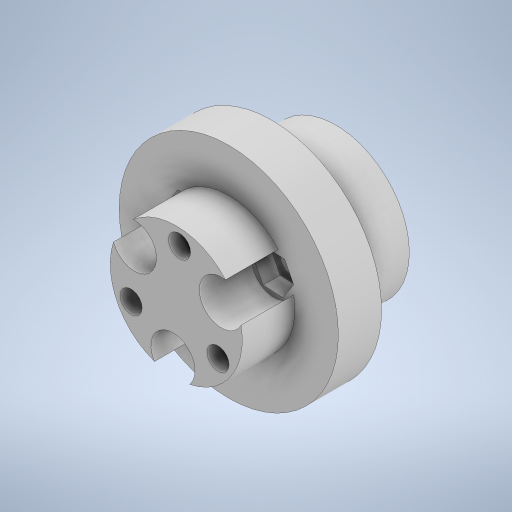
# Autodesk Inventor part: Os
Saved by Autodesk Inventor 2023 (Build 270158000, 158)
## iProperties
Created: 2023-01-20
Part Number: Os
Material: Generic
Document SubType Name: Modeling
Designer: Kamil
Density: 1 g/cm^3
Appearance: Default
Mass: 24.6668 g
Surface Area: 88.8395 cm^2
Volume: 24.6668 cm^3
Author: Kamil
Autodesk Inventor part; units mm, degrees
ref_plane "YZ Plane" through (0, 0, 0) normal (1, 0, 0) x (0, 1, 0)
ref_plane "XZ Plane" through (0, 0, 0) normal (0, 1, 0) x (-1, 0, 0)
ref_plane "XY Plane" through (0, 0, 0) normal (0, 0, 1) x (1, 0, 0)
sketch "Sketch1" plane through (0, 0, 0) normal (0, 0, 1) x (1, 0, 0)
  circle A0 centre (0, 0) radius 23.3333 projected
  arc A1 (-39.2843, 4.1223) -> (-36.4252, -2.8784) centre (-31.328, 3.2874) ccw projected
  arc A2 (-35.6202, -8.1415) -> (-36.4252, -2.8784) centre (-38.9739, -5.9614) ccw projected
  arc A3 (-35.6202, -8.1415) -> (-36.2558, -15.6768) centre (-28.9129, -12.5018) ccw projected
  arc A4 (-36.2558, -15.6768) -> (33.8969, -20.2792) centre (0, 0) ccw projected
  arc A5 (33.8969, -20.2792) -> (34.2512, -12.7254) centre (27.0317, -16.172) ccw projected
  arc A6 (35.737, -7.6127) -> (34.2512, -12.7254) centre (37.861, -11.0021) ccw projected
  arc A7 (35.737, -7.6127) -> (39.4862, -1.0454) centre (31.489, -0.8337) ccw projected
  arc A8 (39.4862, -1.0454) -> (-39.2843, 4.1223) centre (0, 0) ccw projected
  circle A9 centre (-9.1932, -4.5329) radius 2 projected
  circle A10 centre (9.1932, 4.5329) radius 2 projected
  circle A11 centre (-0.671, -10.228) radius 2 projected
  circle A12 centre (-8.5222, 5.6951) radius 2 projected
  circle A13 centre (0.671, 10.228) radius 2 projected
  circle A14 centre (8.5222, -5.6951) radius 2 projected
  circle A15 centre (0, 0) radius 13.4591 projected
  line L0 (-5.9382, 0.859) -> (-7.1311, 0.7284) projected
  arc A16 (-5.6118, -2.1232) -> (-5.9382, 0.859) centre (0, 0) ccw projected
  line L1 (-6.8047, -2.2538) -> (-5.6118, -2.1232) projected
  line L2 (-7.1311, 0.7284) -> (-6.8047, -2.2538) projected
  line L3 (23.3333, 0) -> (22.3333, 0)
  circle A17 centre (0, 0) radius 22.3333
  circle A18 centre (0, 0) radius 6
  circle A19 centre (16.7628, -26.571) radius 3.75 projected
  circle A20 centre (-29.1794, 11.6435) radius 3.75 projected
  circle A21 centre (2.0567, 31.3493) radius 3.75 projected
  circle A22 centre (-20.0905, -24.1532) radius 3.75 projected
  circle A23 centre (30.4505, 7.7314) radius 3.75 projected
  point P0 (0, 0)
  dimension "d0" = 1
  constraints: 2 coincident, 2 end point, 2 horizontal alignment, 1 horizontal, 6 other
  measures "d0" distance of L3.start L3.end
extrude "Extrusion1" add sketch "Sketch1" along normal blind 3.8 contours A15 | A18 L1 L2 L0 | A16 A18 | A17
sketch "Sketch2" plane through (0, 0, 0) normal (0, 0, -1) x (-1, 0, 0)
  circle A0 centre (0, 0) radius 15 projected
  circle A1 centre (0, 0) radius 22.3333 projected
  circle A2 centre (9.1932, -4.5329) radius 2 projected
  circle A3 centre (-9.1932, 4.5329) radius 2 projected
  circle A4 centre (0.671, -10.228) radius 2 projected
  circle A5 centre (8.5222, 5.6951) radius 2 projected
  circle A6 centre (-0.671, 10.228) radius 2 projected
  circle A7 centre (-8.5222, -5.6951) radius 2 projected
  point P0 (0, 0)
ref_plane "Work Plane1" through (-21.6708, -21.6708, -13) normal (0, 0, -1) x (0, 1, 0)
extrude "Extrusion2" add sketch "Sketch2" along normal up to surface (13 mm away) contours A0
sketch "Sketch3" plane through (0, 0, 3.8) normal (0, 0, 1) x (1, 0, 0)
  point P0 (0, 0)
sketch "Sketch4" plane through (0, 0, -13) normal (0, 0, -1) x (-1, 0, 0)
  circle A0 centre (0, 0) radius 15 projected
  circle A1 centre (-8.5222, -5.6951) radius 2 projected
  circle A2 centre (-0.671, 10.228) radius 2 projected
  circle A3 centre (8.5222, 5.6951) radius 2 projected
  circle A4 centre (0.671, -10.228) radius 2 projected
  circle A5 centre (-9.1932, 4.5329) radius 2 projected
  circle A6 centre (9.1932, -4.5329) radius 2 projected
  line L0 (0, 0) -> (9.1932, -4.5329)
  line L1 (9.1932, -4.5329) -> (12.3324, -6.0807)
  circle A7 centre (9.1932, -4.5329) radius 2 projected
  circle A8 centre (9.1932, -4.5329) radius 3.5
  circle A9 centre (8.5222, 5.6951) radius 3.5
  circle A10 centre (-0.671, 10.228) radius 3.5
  circle A11 centre (-9.1932, 4.5329) radius 3.5
  circle A12 centre (-8.5222, -5.6951) radius 3.5
  circle A13 centre (0.671, -10.228) radius 3.5
  point P0 (0, 0)
  point P1 (11.4322, 7.6398)
  point P2 (-0.9001, 13.7205)
  point P3 (-12.3324, 6.0807)
  point P4 (-11.4322, -7.6398)
  point P5 (0.9001, -13.7205)
  dimension "d5" = 3.5
  dimension "d8" = 360
  constraints: 4 end point, 1 coincident, 1 collinear, 37 other
  measures "d5" distance of L0.end L1.end
extrude "Extrusion3" cut sketch "Sketch4" against normal blind 5 contours A1 | A6 L1 L0 | A6 L0 A8 L1 | L0 L1 A6 | A6 L1 A8 L0 | A10 | A12
sketch "Sketch5" plane through (0, 0, 3.8) normal (0, 0, 1) x (1, 0, 0)
  circle A0 centre (0, 0) radius 22.3333 projected
  circle A1 centre (-9.1932, -4.5329) radius 2 projected
  circle A2 centre (9.1932, 4.5329) radius 2 projected
  circle A3 centre (-0.671, -10.228) radius 2 projected
  circle A4 centre (-8.5222, 5.6951) radius 2 projected
  circle A5 centre (0.671, 10.228) radius 2 projected
  circle A6 centre (8.5222, -5.6951) radius 2 projected
  line L0 (0, 0) -> (-0.671, -10.228)
  circle A7 centre (-0.671, -10.228) radius 2 projected
  line L1 (-0.671, -10.228) -> (-1.462, -22.2854)
  circle A8 centre (0, 0) radius 22.3333 projected
  line L2 (-0.671, -10.228) -> (-0.9001, -13.7205)
  line L3 (-3.0871, -13.8731) -> (-5.0083, -9.9765)
  line L4 (-5.0083, -9.9765) -> (-2.5944, -6.3644)
  line L5 (-2.5944, -6.3644) -> (1.7407, -6.6488)
  line L6 (1.7407, -6.6488) -> (3.662, -10.5454)
  line L7 (3.662, -10.5454) -> (1.2481, -14.1575)
  line L8 (1.2481, -14.1575) -> (-3.0871, -13.8731)
  line L9 (4.2145, -5.429) -> (6.6284, -1.8169)
  line L10 (6.1358, -9.3256) -> (4.2145, -5.429)
  line L11 (10.4709, -9.61) -> (6.1358, -9.3256)
  line L12 (12.8848, -5.9979) -> (10.4709, -9.61)
  line L13 (10.9635, -2.1013) -> (12.8848, -5.9979)
  line L14 (6.6284, -1.8169) -> (10.9635, -2.1013)
  line L15 (6.8089, 0.9353) -> (4.8877, 4.8319)
  line L16 (11.1441, 0.6509) -> (6.8089, 0.9353)
  line L17 (13.558, 4.2631) -> (11.1441, 0.6509)
  line L18 (11.6367, 8.1596) -> (13.558, 4.2631)
  line L19 (7.3016, 8.4441) -> (11.6367, 8.1596)
  line L20 (4.8877, 4.8319) -> (7.3016, 8.4441)
  line L21 (2.5944, 6.3644) -> (-1.7407, 6.6488)
  line L22 (5.0083, 9.9765) -> (2.5944, 6.3644)
  line L23 (3.0871, 13.8731) -> (5.0083, 9.9765)
  line L24 (-1.2481, 14.1575) -> (3.0871, 13.8731)
  line L25 (-3.662, 10.5454) -> (-1.2481, 14.1575)
  line L26 (-1.7407, 6.6488) -> (-3.662, 10.5454)
  line L27 (-4.2145, 5.429) -> (-6.6284, 1.8169)
  line L28 (-6.1358, 9.3256) -> (-4.2145, 5.429)
  line L29 (-10.4709, 9.61) -> (-6.1358, 9.3256)
  line L30 (-12.8848, 5.9979) -> (-10.4709, 9.61)
  line L31 (-10.9635, 2.1013) -> (-12.8848, 5.9979)
  line L32 (-6.6284, 1.8169) -> (-10.9635, 2.1013)
  line L33 (-6.8089, -0.9353) -> (-4.8877, -4.8319)
  line L34 (-11.1441, -0.6509) -> (-6.8089, -0.9353)
  line L35 (-13.558, -4.2631) -> (-11.1441, -0.6509)
  line L36 (-11.6367, -8.1596) -> (-13.558, -4.2631)
  line L37 (-7.3016, -8.4441) -> (-11.6367, -8.1596)
  line L38 (-4.8877, -4.8319) -> (-7.3016, -8.4441)
  point P0 (0, 0)
  point P1 (-0.6732, -10.261)
  point P2 (-0.9195, -14.0153)
  point P3 (11.6779, -7.8039)
  point P4 (12.5974, 6.2114)
  point P5 (0.9195, 14.0153)
  point P6 (-11.6779, 7.8039)
  point P7 (-12.5974, -6.2114)
  dimension "d13" = 3.5
  dimension "d16" = 360
  constraints: 78 end point, 2 point on line, 1 collinear, 1 midpoint, 94 other
  measures "d13" distance of L1.start L2.end
extrude "Extrusion4" add sketch "Sketch5" along normal blind 5 contours A0 | L9 L14 L13 L12 L11 L10 | L21 L26 L25 L24 L23 L22 | L33 L38 L37 L36 L35 L34
sketch "Sketch6" plane through (0, 0, 3.8) normal (0, 0, 1) x (1, 0, 0)
  line L0 (6.8089, 0.9353) -> (11.1441, 0.6509) projected
  line L1 (11.1441, 0.6509) -> (13.558, 4.2631) projected
  line L2 (13.558, 4.2631) -> (11.6367, 8.1596) projected
  line L3 (11.6367, 8.1596) -> (7.3016, 8.4441) projected
  line L4 (7.3016, 8.4441) -> (4.8877, 4.8319) projected
  line L5 (4.8877, 4.8319) -> (6.8089, 0.9353) projected
  circle A0 centre (9.1932, 4.5329) radius 2 projected
  circle A1 centre (0, 0) radius 22.3333 projected
  circle A2 centre (8.5222, -5.6951) radius 2 projected
  circle A3 centre (0.671, 10.228) radius 2 projected
  circle A4 centre (-9.1932, -4.5329) radius 2 projected
  line L6 (1.2481, -14.1575) -> (-3.0871, -13.8731) projected
  line L7 (-3.0871, -13.8731) -> (-5.0083, -9.9765) projected
  line L8 (-5.0083, -9.9765) -> (-2.5944, -6.3644) projected
  line L9 (-2.5944, -6.3644) -> (1.7407, -6.6488) projected
  line L10 (1.7407, -6.6488) -> (3.662, -10.5454) projected
  line L11 (3.662, -10.5454) -> (1.2481, -14.1575) projected
  line L12 (-4.2145, 5.429) -> (-6.6284, 1.8169) projected
  line L13 (-6.6284, 1.8169) -> (-10.9635, 2.1013) projected
  line L14 (-10.9635, 2.1013) -> (-12.8848, 5.9979) projected
  line L15 (-12.8848, 5.9979) -> (-10.4709, 9.61) projected
  line L16 (-10.4709, 9.61) -> (-6.1358, 9.3256) projected
  line L17 (-6.1358, 9.3256) -> (-4.2145, 5.429) projected
  line L18 (6.8089, 0.9353) -> (4.8877, 4.8319) projected
  line L19 (4.8877, 4.8319) -> (7.3016, 8.4441) projected
  line L20 (7.3016, 8.4441) -> (11.6367, 8.1596) projected
  line L21 (11.6367, 8.1596) -> (13.558, 4.2631) projected
  line L22 (13.558, 4.2631) -> (11.1441, 0.6509) projected
  line L23 (11.1441, 0.6509) -> (6.8089, 0.9353) projected
  circle A5 centre (-0.671, -10.228) radius 2 projected
  circle A6 centre (-8.5222, 5.6951) radius 2 projected
  point P0 (0, 0)
extrude "Extrusion5" add sketch "Sketch6" along normal blind 1.5 contours L5 L4 L3 L2 L1 L0 | L6 L7 L8 L9 L10 L11 | L12 L13 L14 L15 L16 L17
sketch "Sketch7" plane through (0, 0, 8.8) normal (0, 0, 1) x (1, 0, 0)
  circle A0 centre (8.5222, -5.6951) radius 2 projected
  circle A1 centre (9.1932, 4.5329) radius 2 projected
  circle A2 centre (-0.671, -10.228) radius 2 projected
  circle A3 centre (0.671, 10.228) radius 2 projected
  circle A4 centre (-9.1932, -4.5329) radius 2 projected
  arc A5 (5.9995, 0.0758) -> (5.2863, -2.8382) centre (0, 0) ccw projected
  line L0 (7.1651, -0.2095) -> (5.9995, 0.0758) projected
  line L1 (6.4519, -3.1235) -> (7.1651, -0.2095) projected
  line L2 (5.2863, -2.8382) -> (6.4519, -3.1235) projected
  circle A6 centre (-8.5222, 5.6951) radius 2 projected
  circle A7 centre (0, 0) radius 13.4542 projected
  circle A8 centre (0, 0) radius 6
  circle A9 centre (0, 0) radius 22.3333 projected
  circle A10 centre (8.5222, -5.6951) radius 2 projected
  circle A11 centre (0.671, 10.228) radius 2 projected
  circle A12 centre (-9.1932, -4.5329) radius 2 projected
  line L3 (1.2481, -14.1575) -> (-3.0871, -13.8731) projected
  line L4 (-3.0871, -13.8731) -> (-5.0083, -9.9765) projected
  line L5 (-5.0083, -9.9765) -> (-2.5944, -6.3644) projected
  line L6 (-2.5944, -6.3644) -> (1.7407, -6.6488) projected
  line L7 (1.7407, -6.6488) -> (3.662, -10.5454) projected
  line L8 (3.662, -10.5454) -> (1.2481, -14.1575) projected
  line L9 (-4.2145, 5.429) -> (-6.6284, 1.8169) projected
  line L10 (-6.6284, 1.8169) -> (-10.9635, 2.1013) projected
  line L11 (-10.9635, 2.1013) -> (-12.8848, 5.9979) projected
  line L12 (-12.8848, 5.9979) -> (-10.4709, 9.61) projected
  line L13 (-10.4709, 9.61) -> (-6.1358, 9.3256) projected
  line L14 (-6.1358, 9.3256) -> (-4.2145, 5.429) projected
  line L15 (6.8089, 0.9353) -> (4.8877, 4.8319) projected
  line L16 (4.8877, 4.8319) -> (7.3016, 8.4441) projected
  line L17 (7.3016, 8.4441) -> (11.6367, 8.1596) projected
  line L18 (11.6367, 8.1596) -> (13.558, 4.2631) projected
  line L19 (13.558, 4.2631) -> (11.1441, 0.6509) projected
  line L20 (11.1441, 0.6509) -> (6.8089, 0.9353) projected
  point P0 (0, 0)
  point P1 (1.7989, -13.3334)
  point P2 (13.0072, 3.4389)
  point P3 (10.6476, 8.2245)
  point P4 (-9.4818, 9.5451)
  point P5 (-12.4465, 5.1088)
  point P6 (-3.5254, -12.9841)
  point P7 (5.9995, 0.0758)
  constraints: 1 coincident, 3 other
extrude "Extrusion6" add sketch "Sketch7" along normal blind 5.2 contours L0 L1 L2 A8 | A7 L8 L7 L6 L5 L4 L11 L10 L9 L14 L13 L17 L16 L15 L20 L19
sketch "Sketch8" plane through (0, 0, 8.8) normal (0, 0, 1) x (1, 0, 0)
  circle A0 centre (0, 0) radius 6 projected
  point P0 (0, 0)
extrude "Extrusion7" add sketch "Sketch8" along normal up to surface (5.2 mm away)
sketch "Sketch9" plane through (0, 0, 14) normal (0, 0, 1) x (1, 0, 0)
  line L0 (3.662, -10.5454) -> (1.7989, -13.3334) projected
  arc A0 (1.7989, -13.3334) -> (13.0072, 3.4389) centre (0, 0) ccw projected
  line L1 (13.0072, 3.4389) -> (11.1441, 0.6509) projected
  line L2 (11.1441, 0.6509) -> (6.8089, 0.9353) projected
  line L3 (6.8089, 0.9353) -> (4.8877, 4.8319) projected
  line L4 (4.8877, 4.8319) -> (7.3016, 8.4441) projected
  line L5 (7.3016, 8.4441) -> (10.6476, 8.2245) projected
  arc A1 (10.6476, 8.2245) -> (-9.4818, 9.5451) centre (0, 0) ccw projected
  line L6 (-9.4818, 9.5451) -> (-6.1358, 9.3256) projected
  line L7 (-6.1358, 9.3256) -> (-4.2145, 5.429) projected
  line L8 (-4.2145, 5.429) -> (-6.6284, 1.8169) projected
  line L9 (-6.6284, 1.8169) -> (-10.9635, 2.1013) projected
  line L10 (-10.9635, 2.1013) -> (-12.4465, 5.1088) projected
  arc A2 (-12.4465, 5.1088) -> (-3.5254, -12.9841) centre (0, 0) ccw projected
  line L11 (-3.5254, -12.9841) -> (-5.0083, -9.9765) projected
  line L12 (-5.0083, -9.9765) -> (-2.5944, -6.3644) projected
  line L13 (-2.5944, -6.3644) -> (1.7407, -6.6488) projected
  line L14 (1.7407, -6.6488) -> (3.662, -10.5454) projected
  circle A3 centre (8.5222, -5.6951) radius 2 projected
  circle A4 centre (0.671, 10.228) radius 2 projected
  circle A5 centre (-9.1932, -4.5329) radius 2 projected
  point P0 (0, 0)
extrude "Extrusion8" add sketch "Sketch9" along normal blind 5.5
fillet "Fillet2" radius 0.4 12 edges at (-4.2669, -11.4803, 19.5) (-3.5254, -12.9841, 14.15) (2.7304, -11.9394, 19.5) (1.7989, -13.3334, 14.15) (12.0757, 2.0449, 19.5) (13.0072, 3.4389, 14.15) (8.9746, 8.3343, 19.5) (10.6476, 8.2245, 14.15) (-7.8088, 9.4354, 19.5) (-9.4818, 9.5451, 14.15) (-11.705, 3.6051, 19.5) (-12.4465, 5.1088, 14.15)
sketch "Sketch10" plane through (0, 0, 19.5) normal (0, 0, 1) x (1, 0, 0)
  line L0 (-12.5711, 4.457) -> (-11.4244, 2.1315) projected
  line L1 (-5.265, -10.3606) -> (-4.1183, -12.686) projected
  line L2 (-5.265, -10.3606) -> (-2.5944, -6.3644) projected
  line L3 (-2.5944, -6.3644) -> (1.7407, -6.6488) projected
  line L4 (1.7407, -6.6488) -> (3.8663, -10.9596) projected
  line L5 (2.4256, -13.1154) -> (3.8663, -10.9596) projected
  line L6 (11.605, 0.6207) -> (13.0456, 2.7764) projected
  line L7 (11.605, 0.6207) -> (6.8089, 0.9353) projected
  line L8 (6.8089, 0.9353) -> (4.8877, 4.8319) projected
  line L9 (4.8877, 4.8319) -> (7.5582, 8.8281) projected
  line L10 (10.1454, 8.6583) -> (7.5582, 8.8281) projected
  line L11 (-6.34, 9.7399) -> (-8.9273, 9.9096) projected
  line L12 (-6.34, 9.7399) -> (-4.2145, 5.429) projected
  line L13 (-4.2145, 5.429) -> (-6.6284, 1.8169) projected
  line L14 (-6.6284, 1.8169) -> (-11.4244, 2.1315) projected
  circle A0 centre (-9.1932, -4.5329) radius 2 projected
  circle A1 centre (0.671, 10.228) radius 2 projected
  circle A2 centre (8.5222, -5.6951) radius 2 projected
  circle A3 centre (-8.5222, 5.6951) radius 2 projected
  circle A4 centre (-0.671, -10.228) radius 2 projected
  circle A5 centre (9.1932, 4.5329) radius 2 projected
  circle A6 centre (-8.5222, 5.6951) radius 2.25
  circle A7 centre (0.671, 10.228) radius 2 projected
  circle A8 centre (0.671, 10.228) radius 2.25
  circle A9 centre (9.1932, 4.5329) radius 2.25
  circle A10 centre (-0.671, -10.228) radius 2.25
  circle A11 centre (8.5222, -5.6951) radius 2 projected
  circle A12 centre (8.5222, -5.6951) radius 2.25
  circle A13 centre (-9.1932, -4.5329) radius 2 projected
  circle A14 centre (-9.1932, -4.5329) radius 2.25
  arc A15 (-12.5711, 4.457) -> (-12.7739, 4.2238) centre (-12.3942, 4.0983) ccw projected
  arc A16 (-12.7739, 4.2238) -> (-4.4268, -12.705) centre (0, 0) ccw projected
  arc A17 (-4.4268, -12.705) -> (-4.1183, -12.686) centre (-4.2952, -12.3273) ccw projected
  arc A18 (2.4256, -13.1154) -> (2.729, -13.1745) centre (2.6479, -12.7828) ccw projected
  arc A19 (2.729, -13.1745) -> (13.2163, 2.5187) centre (0, 0) ccw projected
  arc A20 (13.2163, 2.5187) -> (13.0456, 2.7764) centre (12.8234, 2.4439) ccw projected
  arc A21 (10.1454, 8.6583) -> (10.0449, 8.9506) centre (9.7463, 8.6845) ccw projected
  arc A22 (10.0449, 8.9506) -> (-8.7894, 10.1863) centre (0, 0) ccw projected
  arc A23 (-8.7894, 10.1863) -> (-8.9273, 9.9096) centre (-8.5281, 9.8834) ccw projected
  point P0 (0, 0)
  dimension "d30" = 4.5
  dimension "d31" = 4.5
  dimension "d32" = 4.5
  dimension "d33" = 4.5
  dimension "d34" = 4.5
  dimension "d35" = 4.5
  constraints: 6 centre point, 5 coincident
  measures "d30" diameter of A6
  measures "d31" diameter of A8
  measures "d32" diameter of A9
  measures "d33" diameter of A10
  measures "d34" diameter of A12
  measures "d35" diameter of A14
extrude "Extrusion9" cut sketch "Sketch10" against normal through all contours A0 | A1 | A2 | A3 | A4 | A5 | A6 | A8 | A9 | A10 | A12 | A14
sketch "Sketch12" plane through (-9.1932, -4.5329, -8) normal (0, 0, -1) x (-1, 0, 0)
  circle A0 centre (-8.5222, -5.6951) radius 2.25 projected
  circle A1 centre (-0.671, 10.228) radius 2.25 projected
  circle A2 centre (-18.3864, 9.0658) radius 2.25 projected
  circle A3 centre (-9.8642, 14.7609) radius 3.5 projected
  circle A4 centre (-17.7154, -1.1622) radius 3.5 projected
  circle A5 centre (0, 0) radius 3.5 projected
  circle A6 centre (-9.1932, 4.5329) radius 15 projected
  point P0 (-9.1932, 4.5329)
extrude "Extrusion11" cut sketch "Sketch12" against normal blind 3 contours A3 | A4 | A5
sketch "Szkic15" plane through (0, 0, 5.3) normal (0, 0, 1) x (1, 0, 0)
  circle A0 centre (-8.5222, 5.6951) radius 2.25 projected
  line L0 (-10.4709, 9.61) -> (-6.1358, 9.3256) projected
  line L1 (-12.8848, 5.9979) -> (-10.4709, 9.61) projected
  line L2 (-10.9635, 2.1013) -> (-12.8848, 5.9979) projected
  line L3 (-6.6284, 1.8169) -> (-10.9635, 2.1013) projected
  line L4 (-4.2145, 5.429) -> (-6.6284, 1.8169) projected
  line L5 (-6.1358, 9.3256) -> (-4.2145, 5.429) projected
  circle A1 centre (-0.671, -10.228) radius 2.25 projected
  line L6 (1.7407, -6.6488) -> (3.662, -10.5454) projected
  line L7 (-2.5944, -6.3644) -> (1.7407, -6.6488) projected
  line L8 (-5.0083, -9.9765) -> (-2.5944, -6.3644) projected
  line L9 (-3.0871, -13.8731) -> (-5.0083, -9.9765) projected
  line L10 (1.2481, -14.1575) -> (-3.0871, -13.8731) projected
  line L11 (3.662, -10.5454) -> (1.2481, -14.1575) projected
  circle A2 centre (9.1932, 4.5329) radius 2.25 projected
  line L12 (11.1441, 0.6509) -> (6.8089, 0.9353) projected
  line L13 (13.558, 4.2631) -> (11.1441, 0.6509) projected
  line L14 (11.6367, 8.1596) -> (13.558, 4.2631) projected
  line L15 (7.3016, 8.4441) -> (11.6367, 8.1596) projected
  line L16 (4.8877, 4.8319) -> (7.3016, 8.4441) projected
  line L17 (6.8089, 0.9353) -> (4.8877, 4.8319) projected
  arc A3 (10.0449, 8.9506) -> (-8.7894, 10.1863) centre (0, 0) ccw projected
  arc A4 (9.7201, 8.2854) -> (10.0449, 8.9506) centre (9.7463, 8.6845) ccw projected
  line L18 (9.7201, 8.2854) -> (11.6367, 8.1596) projected
  line L19 (11.6367, 8.1596) -> (13.558, 4.2631) projected
  line L20 (13.558, 4.2631) -> (12.4908, 2.6661) projected
  arc A5 (13.2163, 2.5187) -> (12.4908, 2.6661) centre (12.8234, 2.4439) ccw projected
  arc A6 (2.729, -13.1745) -> (13.2163, 2.5187) centre (0, 0) ccw projected
  arc A7 (2.3153, -12.5605) -> (2.729, -13.1745) centre (2.6479, -12.7828) ccw projected
  line L21 (2.3153, -12.5605) -> (1.2481, -14.1575) projected
  line L22 (1.2481, -14.1575) -> (-3.0871, -13.8731) projected
  line L23 (-3.0871, -13.8731) -> (-3.9365, -12.1504) projected
  arc A8 (-4.4268, -12.705) -> (-3.9365, -12.1504) centre (-4.2952, -12.3273) ccw projected
  arc A9 (-12.7739, 4.2238) -> (-4.4268, -12.705) centre (0, 0) ccw projected
  arc A10 (-12.0354, 4.2751) -> (-12.7739, 4.2238) centre (-12.3942, 4.0983) ccw projected
  line L24 (-12.0354, 4.2751) -> (-12.8848, 5.9979) projected
  line L25 (-12.8848, 5.9979) -> (-10.4709, 9.61) projected
  line L26 (-10.4709, 9.61) -> (-8.5543, 9.4843) projected
  arc A11 (-8.7894, 10.1863) -> (-8.5543, 9.4843) centre (-8.5281, 9.8834) ccw projected
  line L27 (-8.5222, 5.6951) -> (-8.3034, 9.4678)
  line L28 (-8.5222, 5.6951) -> (-8.3195, 9.1892)
  line L29 (-6.3022, 9.0722) -> (-4.4875, 5.4611)
  line L30 (-4.4875, 5.4611) -> (-6.7076, 2.084)
  line L31 (-6.7076, 2.084) -> (-10.7422, 2.318)
  line L32 (-10.7422, 2.318) -> (-12.5569, 5.9292)
  line L33 (-12.5569, 5.9292) -> (-10.3368, 9.3063)
  line L34 (-10.3368, 9.3063) -> (-6.3022, 9.0722)
  line L35 (-13.2279, -4.2988) -> (-11.0079, -0.9217)
  line L36 (-11.0079, -0.9217) -> (-6.9732, -1.1558)
  line L37 (-11.4133, -7.91) -> (-13.2279, -4.2988)
  line L38 (-7.3786, -8.144) -> (-11.4133, -7.91)
  line L39 (-5.1586, -4.767) -> (-7.3786, -8.144)
  line L40 (-6.9732, -1.1558) -> (-5.1586, -4.767)
  line L41 (-2.891, -13.6051) -> (-4.7057, -9.994)
  line L42 (-4.7057, -9.994) -> (-2.4856, -6.6169)
  line L43 (1.1436, -13.8392) -> (-2.891, -13.6051)
  line L44 (3.3637, -10.4621) -> (1.1436, -13.8392)
  line L45 (1.549, -6.8509) -> (3.3637, -10.4621)
  line L46 (-2.4856, -6.6169) -> (1.549, -6.8509)
  line L47 (10.3368, -9.3063) -> (6.3022, -9.0722)
  line L48 (6.3022, -9.0722) -> (4.4875, -5.4611)
  line L49 (12.5569, -5.9292) -> (10.3368, -9.3063)
  line L50 (10.7422, -2.318) -> (12.5569, -5.9292)
  line L51 (6.7076, -2.084) -> (10.7422, -2.318)
  line L52 (4.4875, -5.4611) -> (6.7076, -2.084)
  line L53 (13.2279, 4.2988) -> (11.0079, 0.9217)
  line L54 (11.0079, 0.9217) -> (6.9732, 1.1558)
  line L55 (11.4133, 7.91) -> (13.2279, 4.2988)
  line L56 (7.3786, 8.144) -> (11.4133, 7.91)
  line L57 (5.1586, 4.767) -> (7.3786, 8.144)
  line L58 (6.9732, 1.1558) -> (5.1586, 4.767)
  line L59 (2.891, 13.6051) -> (4.7057, 9.994)
  line L60 (4.7057, 9.994) -> (2.4856, 6.6169)
  line L61 (-1.1436, 13.8392) -> (2.891, 13.6051)
  line L62 (-3.3637, 10.4621) -> (-1.1436, 13.8392)
  line L63 (-1.549, 6.8509) -> (-3.3637, 10.4621)
  line L64 (2.4856, 6.6169) -> (-1.549, 6.8509)
  point P0 (0, 0)
  point P1 (-12.1179, -2.6103)
  point P2 (-3.7984, -11.7995)
  point P3 (8.3195, -9.1892)
  point P4 (12.1179, 2.6103)
  point P5 (3.7984, 11.7995)
  dimension "d54" = 3.5
  constraints: 76 end point, 2 midpoint, 1 coincident, 1 point on line, 13 other
  measures "d54" distance of L27.start L28.end
extrude "Wyciągnięcie proste14" add sketch "Szkic15" along normal up to surface (14.2 mm away) contours L0 L5 L4 L3 L2 L1 | L15 L14 L13 L12 L17 L16 | L9 L8 L7 L6 L11 L10
sketch "Szkic16" plane through (0, 0, 19.5) normal (0, 0, 1) x (1, 0, 0)
  line L0 (13.2279, 4.2988) -> (11.4133, 7.91) projected
  line L1 (11.0079, 0.9217) -> (13.2279, 4.2988) projected
  line L2 (6.9732, 1.1558) -> (11.0079, 0.9217) projected
  line L3 (5.1586, 4.767) -> (6.9732, 1.1558) projected
  line L4 (7.3786, 8.144) -> (5.1586, 4.767) projected
  line L5 (11.4133, 7.91) -> (7.3786, 8.144) projected
  line L6 (-2.891, -13.6051) -> (1.1436, -13.8392) projected
  line L7 (-4.7057, -9.994) -> (-2.891, -13.6051) projected
  line L8 (-2.4856, -6.6169) -> (-4.7057, -9.994) projected
  line L9 (1.549, -6.8509) -> (-2.4856, -6.6169) projected
  line L10 (3.3637, -10.4621) -> (1.549, -6.8509) projected
  line L11 (1.1436, -13.8392) -> (3.3637, -10.4621) projected
  line L12 (-10.3368, 9.3063) -> (-12.5569, 5.9292) projected
  line L13 (-6.3022, 9.0722) -> (-10.3368, 9.3063) projected
  line L14 (-4.4875, 5.4611) -> (-6.3022, 9.0722) projected
  line L15 (-6.7076, 2.084) -> (-4.4875, 5.4611) projected
  line L16 (-10.7422, 2.318) -> (-6.7076, 2.084) projected
  line L17 (-12.5569, 5.9292) -> (-10.7422, 2.318) projected
  circle A0 centre (8.5222, -5.6951) radius 2.25 projected
  line L18 (11.605, 0.6207) -> (13.0456, 2.7764) projected
  line L19 (11.605, 0.6207) -> (11.1441, 0.6509) projected
  line L20 (13.558, 4.2631) -> (11.1441, 0.6509) projected
  line L21 (11.6367, 8.1596) -> (13.558, 4.2631) projected
  line L22 (7.3016, 8.4441) -> (11.6367, 8.1596) projected
  line L23 (7.3016, 8.4441) -> (7.5582, 8.8281) projected
  line L24 (10.1454, 8.6583) -> (7.5582, 8.8281) projected
  circle A1 centre (0.671, 10.228) radius 2.25 projected
  line L25 (-6.34, 9.7399) -> (-8.9273, 9.9096) projected
  line L26 (-6.34, 9.7399) -> (-6.1358, 9.3256) projected
  line L27 (-10.4709, 9.61) -> (-6.1358, 9.3256) projected
  line L28 (-12.8848, 5.9979) -> (-10.4709, 9.61) projected
  line L29 (-10.9635, 2.1013) -> (-12.8848, 5.9979) projected
  line L30 (-10.9635, 2.1013) -> (-11.4244, 2.1315) projected
  line L31 (-12.5711, 4.457) -> (-11.4244, 2.1315) projected
  circle A2 centre (-9.1932, -4.5329) radius 2.25 projected
  line L32 (-5.265, -10.3606) -> (-4.1183, -12.686) projected
  line L33 (-5.265, -10.3606) -> (-5.0083, -9.9765) projected
  line L34 (-3.0871, -13.8731) -> (-5.0083, -9.9765) projected
  line L35 (1.2481, -14.1575) -> (-3.0871, -13.8731) projected
  line L36 (3.662, -10.5454) -> (1.2481, -14.1575) projected
  line L37 (3.662, -10.5454) -> (3.8663, -10.9596) projected
  line L38 (2.4256, -13.1154) -> (3.8663, -10.9596) projected
  arc A3 (10.0449, 8.9506) -> (-8.7894, 10.1863) centre (0, 0) ccw projected
  circle A4 centre (0, 0) radius 18.6652
  arc A5 (-12.5711, 4.457) -> (-12.7739, 4.2238) centre (-12.3942, 4.0983) ccw projected
  arc A6 (-12.7739, 4.2238) -> (-4.4268, -12.705) centre (0, 0) ccw projected
  arc A7 (-4.4268, -12.705) -> (-4.1183, -12.686) centre (-4.2952, -12.3273) ccw projected
  arc A8 (2.4256, -13.1154) -> (2.729, -13.1745) centre (2.6479, -12.7828) ccw projected
  arc A9 (2.729, -13.1745) -> (13.2163, 2.5187) centre (0, 0) ccw projected
  arc A10 (13.2163, 2.5187) -> (13.0456, 2.7764) centre (12.8234, 2.4439) ccw projected
  arc A11 (10.1454, 8.6583) -> (10.0449, 8.9506) centre (9.7463, 8.6845) ccw projected
  arc A12 (10.0449, 8.9506) -> (-8.7894, 10.1863) centre (0, 0) ccw projected
  arc A13 (-8.7894, 10.1863) -> (-8.9273, 9.9096) centre (-8.5281, 9.8834) ccw projected
  point P0 (0, 0)
  constraints: 1 centre point, 1 coincident
extrude "Wyciągnięcie proste15" cut sketch "Szkic16" against normal blind 1 contours L1 L2 L3 L4 L5 L0 | L7 L8 L9 L10 L11 L6 | L13 L14 L15 L16 L17 L12 | A0 | L18 A10 A9 A8 L38 L37 L36 L35 L34 L33 L32 A7 A6 A5 L31 L30 L29 L28 L27 L26 L25 A13 A3 A11 L24 L23 L22 L21 L20 L19 | A1 | A2 | A4
sketch "Szkic17" plane through (0, 0, 18.5) normal (0, 0, 1) x (1, 0, 0)
  line L0 (5.1586, 4.767) -> (6.9732, 1.1558) projected
  line L1 (7.3786, 8.144) -> (5.1586, 4.767) projected
  line L2 (11.4133, 7.91) -> (7.3786, 8.144) projected
  line L3 (13.2279, 4.2988) -> (11.4133, 7.91) projected
  line L4 (11.0079, 0.9217) -> (13.2279, 4.2988) projected
  line L5 (6.9732, 1.1558) -> (11.0079, 0.9217) projected
  line L6 (1.549, -6.8509) -> (-2.4856, -6.6169) projected
  line L7 (3.3637, -10.4621) -> (1.549, -6.8509) projected
  line L8 (1.1436, -13.8392) -> (3.3637, -10.4621) projected
  line L9 (-2.891, -13.6051) -> (1.1436, -13.8392) projected
  line L10 (-4.7057, -9.994) -> (-2.891, -13.6051) projected
  line L11 (-2.4856, -6.6169) -> (-4.7057, -9.994) projected
  line L12 (-10.4709, 9.61) -> (-8.5543, 9.4843) projected
  line L13 (-12.8848, 5.9979) -> (-10.4709, 9.61) projected
  line L14 (-12.0354, 4.2751) -> (-12.8848, 5.9979) projected
  arc A0 (-12.0354, 4.2751) -> (-12.7739, 4.2238) centre (-12.3942, 4.0983) ccw projected
  arc A1 (-12.7739, 4.2238) -> (-4.4268, -12.705) centre (0, 0) ccw projected
  arc A2 (-4.4268, -12.705) -> (-3.9365, -12.1504) centre (-4.2952, -12.3273) ccw projected
  line L15 (-3.0871, -13.8731) -> (-3.9365, -12.1504) projected
  line L16 (1.2481, -14.1575) -> (-3.0871, -13.8731) projected
  line L17 (2.3153, -12.5605) -> (1.2481, -14.1575) projected
  arc A3 (2.3153, -12.5605) -> (2.729, -13.1745) centre (2.6479, -12.7828) ccw projected
  arc A4 (2.729, -13.1745) -> (13.2163, 2.5187) centre (0, 0) ccw projected
  arc A5 (13.2163, 2.5187) -> (12.4908, 2.6661) centre (12.8234, 2.4439) ccw projected
  line L18 (13.558, 4.2631) -> (12.4908, 2.6661) projected
  line L19 (11.6367, 8.1596) -> (13.558, 4.2631) projected
  line L20 (9.7201, 8.2854) -> (11.6367, 8.1596) projected
  arc A6 (9.7201, 8.2854) -> (10.0449, 8.9506) centre (9.7463, 8.6845) ccw projected
  arc A7 (10.0449, 8.9506) -> (-8.7894, 10.1863) centre (0, 0) ccw projected
  arc A8 (-8.7894, 10.1863) -> (-8.5543, 9.4843) centre (-8.5281, 9.8834) ccw projected
  line L21 (-10.7422, 2.318) -> (-6.7076, 2.084) projected
  line L22 (-12.5569, 5.9292) -> (-10.7422, 2.318) projected
  line L23 (-10.3368, 9.3063) -> (-12.5569, 5.9292) projected
  line L24 (-6.3022, 9.0722) -> (-10.3368, 9.3063) projected
  line L25 (-4.4875, 5.4611) -> (-6.3022, 9.0722) projected
  line L26 (-6.7076, 2.084) -> (-4.4875, 5.4611) projected
  circle A9 centre (0.671, 10.228) radius 2.25 projected
  circle A10 centre (-9.1932, -4.5329) radius 2.25 projected
  circle A11 centre (8.5222, -5.6951) radius 2.25 projected
  circle A12 centre (0, 0) radius 13.4542
  point P0 (0, 0)
  point P1 (-4.4268, -12.705)
  point P2 (-3.5254, -12.9841)
  point P3 (1.7989, -13.3334)
  point P4 (2.729, -13.1745)
  point P5 (13.2163, 2.5187)
  point P6 (13.0072, 3.4389)
  point P7 (10.6476, 8.2245)
  point P8 (10.0449, 8.9506)
  point P9 (-12.4465, 5.1088)
  point P10 (-12.7739, 4.2238)
  point P11 (-8.7894, 10.1863)
  point P12 (-9.4818, 9.5451)
  constraints: 1 centre point, 1 coincident
extrude "Wyciągnięcie proste16" add sketch "Szkic17" against normal up to surface (9.7 mm away) contours L20 A6 A12 | A12 A5 L18 | A8 L12 A12 | A12 L17 A3 | L14 A0 A12 | A12 A2 L15
sketch "Szkic18" plane through (0, 0, 18.5) normal (0, 0, 1) x (1, 0, 0)
  line L0 (5.1586, 4.767) -> (6.9732, 1.1558) projected
  line L1 (7.3786, 8.144) -> (5.1586, 4.767) projected
  line L2 (11.4133, 7.91) -> (7.3786, 8.144) projected
  line L3 (13.2279, 4.2988) -> (11.4133, 7.91) projected
  line L4 (11.0079, 0.9217) -> (13.2279, 4.2988) projected
  line L5 (6.9732, 1.1558) -> (11.0079, 0.9217) projected
  line L6 (1.549, -6.8509) -> (-2.4856, -6.6169) projected
  line L7 (3.3637, -10.4621) -> (1.549, -6.8509) projected
  line L8 (1.1436, -13.8392) -> (3.3637, -10.4621) projected
  line L9 (-2.891, -13.6051) -> (1.1436, -13.8392) projected
  line L10 (-4.7057, -9.994) -> (-2.891, -13.6051) projected
  line L11 (-2.4856, -6.6169) -> (-4.7057, -9.994) projected
  line L12 (-10.4709, 9.61) -> (-9.4818, 9.5451) projected
  line L13 (-12.8848, 5.9979) -> (-10.4709, 9.61) projected
  line L14 (-12.4465, 5.1088) -> (-12.8848, 5.9979) projected
  arc A0 (-12.4465, 5.1088) -> (-3.5254, -12.9841) centre (0, 0) ccw projected
  line L15 (-3.0871, -13.8731) -> (-3.5254, -12.9841) projected
  line L16 (1.2481, -14.1575) -> (-3.0871, -13.8731) projected
  line L17 (1.7989, -13.3334) -> (1.2481, -14.1575) projected
  arc A1 (1.7989, -13.3334) -> (13.0072, 3.4389) centre (0, 0) ccw projected
  line L18 (13.558, 4.2631) -> (13.0072, 3.4389) projected
  line L19 (11.6367, 8.1596) -> (13.558, 4.2631) projected
  line L20 (10.6476, 8.2245) -> (11.6367, 8.1596) projected
  arc A2 (10.6476, 8.2245) -> (-9.4818, 9.5451) centre (0, 0) ccw projected
  line L21 (-10.7422, 2.318) -> (-6.7076, 2.084) projected
  line L22 (-12.5569, 5.9292) -> (-10.7422, 2.318) projected
  line L23 (-10.3368, 9.3063) -> (-12.5569, 5.9292) projected
  line L24 (-6.3022, 9.0722) -> (-10.3368, 9.3063) projected
  line L25 (-4.4875, 5.4611) -> (-6.3022, 9.0722) projected
  line L26 (-6.7076, 2.084) -> (-4.4875, 5.4611) projected
  circle A3 centre (0.671, 10.228) radius 2.25 projected
  circle A4 centre (-9.1932, -4.5329) radius 2.25 projected
  circle A5 centre (8.5222, -5.6951) radius 2.25 projected
  circle A6 centre (0, 0) radius 13.4542
  point P0 (0, 0)
  point P1 (12.9044, 3.8067)
  point P2 (13.0072, 3.4389)
  point P3 (10.8599, 7.9421)
  point P4 (-3.1555, -13.0789)
  point P5 (-3.5254, -12.9841)
  point P6 (1.4481, -13.376)
  point P7 (-12.308, 5.4339)
  point P8 (-9.7489, 9.2722)
  constraints: 1 centre point, 1 coincident, 1 concentric
extrude "Wyciągnięcie proste17" cut sketch "Szkic18" against normal up to surface (9.7 mm away) contours A6 L20 L19 L18 L4 L3 L2 | A6 L24 L23 L22 L14 L13 L12 | L17 L16 L15 A6 L10 L9 L8
sketch "Szkic19" plane through (0, 0, 18.5) normal (0, 0, 1) x (1, 0, 0)
  circle A0 centre (8.5222, -5.6951) radius 2.25 projected
  circle A1 centre (-9.1932, -4.5329) radius 2.25 projected
  circle A2 centre (0.671, 10.228) radius 2.25 projected
  arc A3 (1.4481, -13.376) -> (12.9044, 3.8067) centre (0, 0) ccw projected
  line L0 (11.0079, 0.9217) -> (12.9044, 3.8067) projected
  line L1 (6.9732, 1.1558) -> (11.0079, 0.9217) projected
  line L2 (5.1586, 4.767) -> (6.9732, 1.1558) projected
  line L3 (7.3786, 8.144) -> (5.1586, 4.767) projected
  line L4 (10.8599, 7.9421) -> (7.3786, 8.144) projected
  arc A4 (10.8599, 7.9421) -> (-9.7489, 9.2722) centre (0, 0) ccw projected
  line L5 (-6.3022, 9.0722) -> (-9.7489, 9.2722) projected
  line L6 (-4.4875, 5.4611) -> (-6.3022, 9.0722) projected
  line L7 (-6.7076, 2.084) -> (-4.4875, 5.4611) projected
  line L8 (-10.7422, 2.318) -> (-6.7076, 2.084) projected
  line L9 (-12.308, 5.4339) -> (-10.7422, 2.318) projected
  arc A5 (-12.308, 5.4339) -> (-3.1555, -13.0789) centre (0, 0) ccw projected
  line L10 (-4.7057, -9.994) -> (-3.1555, -13.0789) projected
  line L11 (-2.4856, -6.6169) -> (-4.7057, -9.994) projected
  line L12 (1.549, -6.8509) -> (-2.4856, -6.6169) projected
  line L13 (3.3637, -10.4621) -> (1.549, -6.8509) projected
  line L14 (1.4481, -13.376) -> (3.3637, -10.4621) projected
  point P0 (0, 0)
extrude "Wyciągnięcie proste18" add sketch "Szkic19" along normal blind 1
sketch "Szkic20" plane through (8.5222, -5.6951, -5) normal (0, 0, -1) x (-1, 0, 0)
  circle A0 centre (0, 0) radius 2.25 projected
  circle A1 centre (0, 0) radius 3.5 projected
  circle A2 centre (7.8512, 15.9231) radius 2.25 projected
  circle A3 centre (7.8512, 15.9231) radius 3.5 projected
  circle A4 centre (17.7154, 1.1622) radius 2.25 projected
  circle A5 centre (17.7154, 1.1622) radius 3.5 projected
  point P0 (8.5222, 5.6951)
extrude "Wyciągnięcie proste19" add sketch "Szkic20" along normal blind 3
sketch "Szkic21" plane through (0, 0, -13) normal (0, 0, -1) x (-1, 0, 0)
  circle A0 centre (0.671, -10.228) radius 2.25 projected
  circle A1 centre (8.5222, 5.6951) radius 2.25 projected
  circle A2 centre (-9.1932, 4.5329) radius 2.25 projected
  circle A3 centre (-0.671, 10.228) radius 3.5 projected
  circle A4 centre (-8.5222, -5.6951) radius 3.5 projected
  circle A5 centre (9.1932, -4.5329) radius 3.5 projected
  circle A6 centre (0, 0) radius 15 projected
  circle A7 centre (-8.5222, -5.6951) radius 3.75
  circle A8 centre (-0.671, 10.228) radius 3.75
  circle A9 centre (9.1932, -4.5329) radius 3.75
  point P0 (0, 0)
  dimension "d82" = 7.5
  dimension "d83" = 7.5
  dimension "d84" = 7.5
  constraints: 3 centre point, 3 coincident
  measures "d82" diameter of A7
  measures "d83" diameter of A8
  measures "d84" diameter of A9
extrude "Wyciągnięcie proste20" cut sketch "Szkic21" against normal up to surface (5 mm away) contours A3 | A4 | A5 | A7 | A8 | A9
sketch "Szkic22" plane through (0, 0, 19.5) normal (0, 0, 1) x (1, 0, 0)
  circle A0 centre (9.1932, 4.5329) radius 2.25 projected
  circle A1 centre (-8.5222, 5.6951) radius 2.25 projected
  circle A2 centre (-9.1932, -4.5329) radius 2.25 projected
  arc A3 (-12.308, 5.4339) -> (-3.1555, -13.0789) centre (0, 0) ccw projected
  circle A4 centre (-0.671, -10.228) radius 2.25 projected
  circle A5 centre (9.1932, 4.5329) radius 4.5
  circle A6 centre (-0.671, -10.228) radius 4.5
  circle A7 centre (-8.5222, 5.6951) radius 4.5
  point P0 (0, 0)
  dimension "d87" = 9
  dimension "d88" = 9
  dimension "d89" = 9
  constraints: 3 centre point, 3 coincident
  measures "d87" diameter of A5
  measures "d88" diameter of A6
  measures "d89" diameter of A7
extrude "Wyciągnięcie proste21" cut sketch "Szkic22" against normal up to surface (10.7 mm away) contours A0 | A4 | A5 | A6 | A7
body "Solid1"
